Autodesk Fusion 360 part; units mm, degrees
note: some values were not read from the file. Chosen so that the rebuilt part matches the saved one: which bodies a step acts on. Set by a fixed rule: which sketch regions a step uses.
(part 5 of 5)
sketch "Sketch3 (7)" plane through (0, 0, -49) normal (0, 0, -1) x (1, 0, 0) in component "backing_ply"
  circle A0 centre (-129.840277, 129.840277) radius 1.6
  circle A1 centre (129.840277, -129.840277) radius 1.6
  circle A2 centre (129.840277, 129.840277) radius 1.6
  circle A3 centre (-129.840277, -129.840277) radius 1.6
  line L0 (143.5, -143.5) -> (143.5, 143.5)
  line L1 (143.5, 143.5) -> (-143.5, 143.5)
  line L2 (-143.5, 143.5) -> (-143.5, -143.5)
  line L3 (-143.5, -143.5) -> (143.5, -143.5)
  circle A4 centre (61.125, 122.25) radius 1.6
  line L4 (53.825, 131.25) -> (53.825, 122.25)
  arc A5 (53.825, 122.25) -> (68.425, 122.25) centre (61.125, 122.25) ccw
  line L5 (68.425, 122.25) -> (68.425, 131.25)
  arc A6 (67.425, 130.25) -> (68.425, 131.25) centre (67.425, 131.25) ccw
  line L6 (67.425, 130.25) -> (54.825, 130.25)
  arc A7 (53.825, 131.25) -> (54.825, 130.25) centre (54.825, 131.25) ccw
  circle A8 centre (122.25, 61.125) radius 1.6
  line L7 (122.25, 53.825) -> (131.25, 53.825)
  arc A9 (130.25, 54.825) -> (131.25, 53.825) centre (131.25, 54.825) ccw
  line L8 (130.25, 54.825) -> (130.25, 67.425)
  arc A10 (131.25, 68.425) -> (130.25, 67.425) centre (131.25, 67.425) ccw
  line L9 (131.25, 68.425) -> (122.25, 68.425)
  arc A11 (122.25, 68.425) -> (122.25, 53.825) centre (122.25, 61.125) ccw
  line L10 (69.3375, -105.4375) -> (99.8375, -105.4375)
  arc A12 (99.8375, -105.4375) -> (99.8375, -94.2375) centre (99.8375, -99.8375) ccw
  line L11 (99.8375, -94.2375) -> (69.3375, -94.2375)
  arc A13 (69.3375, -94.2375) -> (69.3375, -105.4375) centre (69.3375, -99.8375) ccw
  line L12 (69.3375, -99.8375) -> (99.8375, -99.8375) construction
  line L13 (94.8375, -96.2375) -> (74.3375, -96.2375)
  line L14 (74.3375, -96.2375) -> (74.3375, -103.4375)
  line L15 (74.3375, -103.4375) -> (94.8375, -103.4375)
  line L16 (94.8375, -103.4375) -> (94.8375, -96.2375)
  line L17 (94.8375, -96.2375) -> (74.3375, -103.4375) construction
  line L18 (74.3375, -96.2375) -> (94.8375, -103.4375) construction
  circle A14 centre (122.25, -61.125) radius 1.6
  line L19 (131.25, -53.825) -> (122.25, -53.825)
  arc A15 (122.25, -53.825) -> (122.25, -68.425) centre (122.25, -61.125) ccw
  line L20 (122.25, -68.425) -> (131.25, -68.425)
  arc A16 (130.25, -67.425) -> (131.25, -68.425) centre (131.25, -67.425) ccw
  line L21 (130.25, -67.425) -> (130.25, -54.825)
  arc A17 (131.25, -53.825) -> (130.25, -54.825) centre (131.25, -54.825) ccw
  circle A18 centre (61.125, -122.25) radius 1.6
  line L22 (53.825, -122.25) -> (53.825, -131.25)
  arc A19 (54.825, -130.25) -> (53.825, -131.25) centre (54.825, -131.25) ccw
  line L23 (54.825, -130.25) -> (67.425, -130.25)
  arc A20 (68.425, -131.25) -> (67.425, -130.25) centre (67.425, -131.25) ccw
  line L24 (68.425, -131.25) -> (68.425, -122.25)
  arc A21 (68.425, -122.25) -> (53.825, -122.25) centre (61.125, -122.25) ccw
  line L25 (96.8375, -101.569551) -> (99.8375, -103.301602)
  line L26 (99.8375, -103.301602) -> (102.8375, -101.569551)
  line L27 (102.8375, -101.569551) -> (102.8375, -98.105449)
  line L28 (102.8375, -98.105449) -> (99.8375, -96.373398)
  line L29 (99.8375, -96.373398) -> (96.8375, -98.105449)
  line L30 (96.8375, -98.105449) -> (96.8375, -101.569551)
  line L31 (72.3375, -98.105449) -> (69.3375, -96.373398)
  line L32 (69.3375, -96.373398) -> (66.3375, -98.105449)
  line L33 (66.3375, -98.105449) -> (66.3375, -101.569551)
  line L34 (66.3375, -101.569551) -> (69.3375, -103.301602)
  line L35 (69.3375, -103.301602) -> (72.3375, -101.569551)
  line L36 (72.3375, -101.569551) -> (72.3375, -98.105449)
  line L37 (69.3375, -105.5375) -> (99.8375, -105.5375)
  arc A22 (99.8375, -105.5375) -> (99.8375, -94.1375) centre (99.8375, -99.8375) ccw
  line L38 (99.8375, -94.1375) -> (69.3375, -94.1375)
  arc A23 (69.3375, -94.1375) -> (69.3375, -105.5375) centre (69.3375, -99.8375) ccw
  circle A24 centre (-122.25, -61.125) radius 1.6
  line L39 (-122.25, -53.825) -> (-131.25, -53.825)
  arc A25 (-130.25, -54.825) -> (-131.25, -53.825) centre (-131.25, -54.825) ccw
  line L40 (-130.25, -54.825) -> (-130.25, -67.425)
  arc A26 (-131.25, -68.425) -> (-130.25, -67.425) centre (-131.25, -67.425) ccw
  line L41 (-131.25, -68.425) -> (-122.25, -68.425)
  arc A27 (-122.25, -68.425) -> (-122.25, -53.825) centre (-122.25, -61.125) ccw
  circle A28 centre (-61.125, -122.25) radius 1.6
  line L42 (-53.825, -131.25) -> (-53.825, -122.25)
  arc A29 (-53.825, -122.25) -> (-68.425, -122.25) centre (-61.125, -122.25) ccw
  line L43 (-68.425, -122.25) -> (-68.425, -131.25)
  arc A30 (-67.425, -130.25) -> (-68.425, -131.25) centre (-67.425, -131.25) ccw
  line L44 (-67.425, -130.25) -> (-54.825, -130.25)
  arc A31 (-53.825, -131.25) -> (-54.825, -130.25) centre (-54.825, -131.25) ccw
  line L45 (-131.25, -68.425) -> (-68.425, -131.25) construction
  circle A32 centre (-99.8375, -99.8375) radius 5.35
  line L46 (-75, 143.5) -> (-75, -143.5) construction
  line L47 (75, 143.5) -> (75, -143.5) construction
  line L48 (-75, 108.5) -> (75, 108.5) construction
  line L49 (-75, 88.5) -> (75, 88.5) construction
  line L50 (-75, 58.5) -> (75, 58.5) construction
  circle A33 centre (75, 108.5) radius 5
  circle A34 centre (75, 58.5) radius 5
  line L51 (70.285955, 60.166667) -> (75, 73.5)
  line L52 (75, 73.5) -> (79.714045, 60.166667)
  circle A35 centre (75, 88.5) radius 5 construction
  circle A36 centre (75, 93.5) radius 2.5
  circle A37 centre (75, 83.5) radius 2.5
  line L53 (0, 108.5) -> (0, 58.5) construction
  circle A38 centre (-75, 108.5) radius 5
  circle A39 centre (-75, 93.5) radius 2.5
  circle A40 centre (-75, 83.5) radius 2.5
  line L54 (-75, 73.5) -> (-79.714045, 60.166667)
  line L55 (-70.285955, 60.166667) -> (-75, 73.5)
  circle A41 centre (-75, 58.5) radius 5
  line L56 (0, 108.5) -> (75, 58.5) construction
  line L57 (37.5, 83.5) -> (37.5, 108.5) construction
  circle A42 centre (0, 108.5) radius 5
  circle A43 centre (0, 93.5) radius 2.5
  circle A44 centre (0, 83.5) radius 2.5
  line L58 (4.714045, 60.166667) -> (0, 73.5)
  line L59 (0, 73.5) -> (-4.714045, 60.166667)
  circle A45 centre (0, 58.5) radius 5
  line L60 (68.425, -131.25) -> (131.25, -68.425) construction
  point P0 (84.5875, -99.8375)
  point P1 (84.5875, -99.8375)
  point P2 (84.5875, -99.8375)
  point P3 (84.5875, -99.8375)
  point P4 (99.8375, -99.8375)
  point P5 (69.3375, -99.8375)
  point P6 (0, 143.5)
  point P7 (75, 103.5)
  point P8 (99.8375, -99.8375)
  point P9 (72.3375, -99.8375)
  dimension "d403" = 7.2
  dimension "d404" = 20.5
  dimension "d405" = 2
  dimension "d406" = 3
  dimension "d407" = 3
  dimension "d408" = 2
  dimension "d409" = 0.1
  dimension "d410" = 10.7
  dimension "d413" = 150
  dimension "d414" = 75
  dimension "d415" = 10
  dimension "d416" = 10
  dimension "d417" = 10
  dimension "d418" = 15
  dimension "d419" = 5
  dimension "d420" = 5
  dimension "d421" = 35
  dimension "d422" = 50
  dimension "d424" = 30
  dimension "d425" = 15
  constraint tangent L10 A12
  constraint tangent A12 L11
  constraint parallel L10 L11
  constraint tangent L11 A13
  constraint tangent L10 A13
  constraint horizontal L12
  constraint coincident P3 P2
  constraint midpoint L12 P3
  constraint horizontal L13
  constraint perpendicular L13 L14
  constraint parallel L13 L15
  constraint parallel L14 L16
  constraint coincident L17 P3
  constraint coincident L18 P3
  constraint coincident P8 P4
  constraint coincident P5 A13.centre
  constraint coincident A26.start L41.start
  constraint coincident L43.end A30.end
  constraint midpoint L45 A32.centre
  constraint coincident L1 L46.start
  constraint coincident L3 L46.end
  constraint perpendicular L3 L46
  constraint coincident L1 L47.start
  constraint coincident L3 L47.end
  constraint perpendicular L3 L47
  constraint midpoint L1 P6
  constraint coincident L46 L48.start
  constraint coincident L47 L48.end
  constraint perpendicular L47 L48
  constraint coincident L46 L49.start
  constraint coincident L47 L49.end
  constraint perpendicular L47 L49
  constraint coincident L46 L50.start
  constraint coincident L47 L50.end
  constraint perpendicular L47 L50
  constraint coincident L48.end A33.centre
  constraint coincident L50.end A34.centre
  constraint coincident L47 L51.end
  constraint tangent A34 L51
  constraint tangent A34 L52
  constraint coincident L49.end A35.centre
  constraint coincident A35 A36.centre
  constraint coincident L47 A36.centre
  constraint coincident L47 A37.centre
  constraint coincident A35 A37.centre
  constraint coincident A33 P7
  constraint coincident L47 P7
  constraint midpoint L48 L53.start
  constraint midpoint L50 L53.end
  constraint symmetric A33 L53 A38
  constraint symmetric A34 L53 A41
  constraint symmetric L51.end L53 L54.start
  constraint symmetric A36 L53 A39
  constraint symmetric A37 L53 A40
  constraint midpoint L56 L57.start
  constraint coincident L48 L57.end
  constraint perpendicular L48 L57
  constraint symmetric A33 L57 A42
  constraint symmetric A34 L57 A45
  constraint symmetric L51.end L57 L58.end
  constraint symmetric A36 L57 A43
  constraint symmetric A37 L57 A44
  constraint coincident A20.start L24.start
  constraint coincident L20.end A16.end
  constraint midpoint L60 P8
  constraint midpoint L36 P9
  constraint coincident L12 P9
  measures "d403" distance of L13.start L15.end
  measures "d404" distance of L14 L16
  measures "d405" distance of L11 L13
  measures "d406" distance of P8 L30
  measures "d407" distance of P5 L36
  measures "d408" distance of L16 L30
  measures "d410" diameter of A32
  measures "d413" distance of L46 L47
  measures "d414" distance of L47 P6
  measures "d415" diameter of A33
  measures "d416" diameter of A34
  measures "d417" diameter of A35
  measures "d418" distance of L50.end L51.end
  measures "d419" diameter of A36
  measures "d420" diameter of A37
  measures "d421" distance of L1 L48
  measures "d422" distance of L48 L50
  measures "d424" distance of L51.end P7
  measures "d425" distance of L49.end P7
extrude "Extrude3''''''" cut sketch "Sketch3 (7)" against normal blind 10 contours L10 A12 L11 A13 | L13 L14 L15 L16 | L25 L26 L27 L28 L29 L30 | L31 L32 L33 L34 L35 L36 | L37 A22 L38 A23 | A32 | A33 | A34 | A34 L51 L52 | A36 | A37 | A38 | A39 | A40 | L54 L55 A41 | A41 | A42 | A43 | A44 | L58 L59 A45 | A45 picked at (88.004167, -94.904167) picked at (81.170833, -98.6375) picked at (100.8375, -100.41485) picked at (68.3375, -99.26015) picked at (79.504167, -105.470833) picked at (-98.230772, -100.611259) picked at (76.446185, 108.980285) picked at (75.428311, 60.054771) picked at (75, 66.824599) picked at (76.760267, 93.305637) picked at (76.760267, 83.305637) picked at (-73.553815, 108.980285) picked at (-73.239733, 93.305637) picked at (-73.239733, 83.305637) picked at (-75, 66.824599) picked at (-71.930398, 57.383078) picked at (-1.574006, 108.257145) picked at (-0.062275, 94.331003) picked at (-1.856006, 82.886176) picked at (0, 66.824599) picked at (1.18045, 60.362306) bodies 49 in component "backing_ply"
sketch "Sketch1 (6)" plane through (0, 0, -49) normal (0, 0, -1) x (1, 0, 0) in component "programming-port_3d"
  circle A0 centre (75, 83.5) radius 2.5
  circle A1 centre (0, 93.5) radius 2.5
  circle A2 centre (-75, 83.5) radius 2.5
  circle A3 centre (-99.8375, -99.8375) radius 5.35
  circle A4 centre (-75, 93.5) radius 2.5
  circle A5 centre (0, 83.5) radius 2.5
  circle A6 centre (75, 93.5) radius 2.5
  line L0 (75, 73.5) -> (79.714045, 60.166667)
  arc A7 (70.285955, 60.166667) -> (79.714045, 60.166667) centre (75, 58.5) ccw
  line L1 (70.285955, 60.166667) -> (75, 73.5)
  circle A8 centre (0, 108.5) radius 5
  line L2 (-75, 73.5) -> (-70.285955, 60.166667)
  arc A9 (-79.714045, 60.166667) -> (-70.285955, 60.166667) centre (-75, 58.5) ccw
  line L3 (-79.714045, 60.166667) -> (-75, 73.5)
  line L4 (99.8375, -105.5375) -> (69.3375, -105.5375)
  arc A10 (69.3375, -94.1375) -> (69.3375, -105.5375) centre (69.3375, -99.8375) ccw
  line L5 (69.3375, -94.1375) -> (99.8375, -94.1375)
  arc A11 (99.8375, -105.5375) -> (99.8375, -94.1375) centre (99.8375, -99.8375) ccw
  circle A12 centre (-75, 108.5) radius 5
  line L6 (0, 73.5) -> (4.714045, 60.166667)
  arc A13 (-4.714045, 60.166667) -> (4.714045, 60.166667) centre (0, 58.5) ccw
  line L7 (-4.714045, 60.166667) -> (0, 73.5)
  circle A14 centre (75, 108.5) radius 5
  circle A15 centre (-129.840277, 129.840277) radius 1.6
  circle A16 centre (129.840277, -129.840277) radius 1.6
  circle A17 centre (129.840277, 129.840277) radius 1.6
  circle A18 centre (-129.840277, -129.840277) radius 1.6
  line L8 (143.5, -143.5) -> (143.5, 143.5)
  line L9 (143.5, 143.5) -> (-143.5, 143.5)
  line L10 (-143.5, 143.5) -> (-143.5, -143.5)
  line L11 (-143.5, -143.5) -> (143.5, -143.5)
  arc A19 (69.3375, -94.2375) -> (69.3375, -105.4375) centre (69.3375, -99.8375) ccw
  line L12 (99.8375, -94.2375) -> (69.3375, -94.2375)
  line L13 (69.3375, -96.373398) -> (66.3375, -98.105449)
  line L14 (72.3375, -98.105449) -> (69.3375, -96.373398)
  line L15 (66.3375, -98.105449) -> (66.3375, -101.569551)
  line L16 (66.3375, -101.569551) -> (69.3375, -103.301602)
  line L17 (69.3375, -103.301602) -> (72.3375, -101.569551)
  line L18 (72.3375, -101.569551) -> (72.3375, -98.105449)
  line L19 (94.8375, -96.2375) -> (74.3375, -96.2375)
  line L20 (74.3375, -96.2375) -> (74.3375, -103.4375)
  line L21 (74.3375, -103.4375) -> (94.8375, -103.4375)
  line L22 (94.8375, -103.4375) -> (94.8375, -96.2375)
  line L23 (99.8375, -96.373398) -> (96.8375, -98.105449)
  line L24 (102.8375, -98.105449) -> (99.8375, -96.373398)
  line L25 (102.8375, -101.569551) -> (102.8375, -98.105449)
  line L26 (99.8375, -103.301602) -> (102.8375, -101.569551)
  line L27 (96.8375, -101.569551) -> (99.8375, -103.301602)
  line L28 (96.8375, -98.105449) -> (96.8375, -101.569551)
  arc A20 (99.8375, -105.4375) -> (99.8375, -94.2375) centre (99.8375, -99.8375) ccw
  line L29 (69.3375, -105.4375) -> (99.8375, -105.4375)
  line L30 (69.3375, -106.9375) -> (99.8375, -106.9375)
  arc A21 (99.8375, -106.9375) -> (99.8375, -92.7375) centre (99.8375, -99.8375) ccw
  line L31 (99.8375, -92.7375) -> (69.3375, -92.7375)
  arc A22 (69.3375, -92.7375) -> (69.3375, -106.9375) centre (69.3375, -99.8375) ccw
  line L32 (74.3375, -96.2375) -> (94.8375, -103.4375) construction
  line L33 (94.8375, -96.2375) -> (74.3375, -103.4375) construction
  line L34 (78.4875, -103.0875) -> (90.6875, -103.0875)
  arc A23 (90.6875, -103.0875) -> (90.6875, -96.5875) centre (90.6875, -99.8375) ccw
  line L35 (90.6875, -96.5875) -> (78.4875, -96.5875)
  arc A24 (78.4875, -96.5875) -> (78.4875, -103.0875) centre (78.4875, -99.8375) ccw
  line L36 (78.4875, -99.8375) -> (90.6875, -99.8375) construction
  point P0 (84.5875, -99.8375)
  dimension "d426" = 1.5
  dimension "d427" = 12.2
  dimension "d428" = 6.5
  constraint coincident L19.end L20.start
  constraint coincident L21.end L22.start
  constraint coincident L19.start L22.end
  constraint coincident L20.end L21.start
  constraint tangent L34 A23
  constraint tangent A23 L35
  constraint parallel L34 L35
  constraint tangent L35 A24
  constraint tangent L34 A24
  constraint horizontal L36
  constraint midpoint L32 P0
  constraint midpoint L36 P0
  measures "d427" distance of A23.end L35.end
  measures "d428" distance of L34 L35
extrude "Extrude1'''''''" add sketch "Sketch1 (6)" along normal blind 2 separate body contours L4 A10 L5 A11 | A19 L12 A20 L29 | L13 L14 L15 L16 L17 L18 | L19 L20 L21 L22 | L23 L24 L25 L26 L27 L28 | L30 A21 L31 A22 picked at (79.504167, -105.470833) picked at (81.170833, -94.904167) picked at (68.3375, -99.26015) picked at (94.534471, -99.756542) picked at (100.8375, -99.26015) picked at (89.670833, -93.204167) makes body 50 in component "programming-port_3d"
fillet "Fillet1''" radius 1.5 4 edges at (93.9375, 99.8375, -51) (84.5875, 103.0875, -51) (75.2375, 99.8375, -51) (84.5875, 96.5875, -51) on bodies 50 in component "programming-port_3d"
extrude "Extrude2'''''" add sketch "Sketch1 (6)" against normal blind 3 contours A19 L12 A20 L29 picked at (81.170833, -94.904167) bodies 50 in component "programming-port_3d"
sketch "Sketch4 (4)" plane through (0, 0, -46) normal (0, 0, 1) x (-1, 0, 0) in component "programming-port_3d"
  line L0 (-72.3375, -101.569551) -> (-72.3375, -98.105449)
  line L1 (-72.3375, -98.105449) -> (-69.3375, -96.373398)
  line L2 (-69.3375, -96.373398) -> (-66.3375, -98.105449)
  line L3 (-66.3375, -98.105449) -> (-66.3375, -101.569551)
  line L4 (-66.3375, -101.569551) -> (-69.3375, -103.301602)
  line L5 (-69.3375, -103.301602) -> (-72.3375, -101.569551)
  line L6 (-94.8375, -103.4375) -> (-94.8375, -96.2375)
  line L7 (-94.8375, -96.2375) -> (-74.3375, -96.2375)
  line L8 (-74.3375, -96.2375) -> (-74.3375, -103.4375)
  line L9 (-74.3375, -103.4375) -> (-94.8375, -103.4375)
  line L10 (-96.8375, -98.105449) -> (-96.8375, -101.569551)
  line L11 (-96.8375, -101.569551) -> (-99.8375, -103.301602)
  line L12 (-99.8375, -103.301602) -> (-102.8375, -101.569551)
  line L13 (-102.8375, -101.569551) -> (-102.8375, -98.105449)
  line L14 (-102.8375, -98.105449) -> (-99.8375, -96.373398)
  line L15 (-99.8375, -96.373398) -> (-96.8375, -98.105449)
  line L16 (-99.8375, -105.4375) -> (-69.3375, -105.4375)
  arc A0 (-69.3375, -105.4375) -> (-69.3375, -94.2375) centre (-69.3375, -99.8375) ccw
  line L17 (-69.3375, -94.2375) -> (-99.8375, -94.2375)
  arc A1 (-99.8375, -94.2375) -> (-99.8375, -105.4375) centre (-99.8375, -99.8375) ccw
  line L18 (-72.3375, -101.569551) -> (-69.3375, -103.301602)
  line L19 (-69.3375, -103.301602) -> (-66.3375, -101.569551)
  line L20 (-66.3375, -101.569551) -> (-66.3375, -98.105449)
  line L21 (-66.3375, -98.105449) -> (-69.3375, -96.373398)
  line L22 (-69.3375, -96.373398) -> (-72.3375, -98.105449)
  line L23 (-72.3375, -98.105449) -> (-72.3375, -101.569551)
  line L24 (-96.8375, -98.105449) -> (-99.8375, -96.373398)
  line L25 (-99.8375, -96.373398) -> (-102.8375, -98.105449)
  line L26 (-102.8375, -98.105449) -> (-102.8375, -101.569551)
  line L27 (-102.8375, -101.569551) -> (-99.8375, -103.301602)
  line L28 (-99.8375, -103.301602) -> (-96.8375, -101.569551)
  line L29 (-96.8375, -101.569551) -> (-96.8375, -98.105449)
  line L30 (-99.8375, -96.373398) -> (-99.8375, -103.301602) construction
  line L31 (-96.8375, -98.105449) -> (-102.8375, -101.569551) construction
  line L32 (-69.3375, -96.373398) -> (-69.3375, -103.301602) construction
  line L33 (-66.3375, -98.105449) -> (-72.3375, -101.569551) construction
  circle A2 centre (-69.3375, -99.8375) radius 1.6
  circle A3 centre (-99.8375, -99.8375) radius 1.6
  dimension "d437" = 3.2
  dimension "d438" = 3.2
  constraint concentric A0 A2
  constraint concentric A1 A3
  measures "d437" diameter of A2
  measures "d438" diameter of A3
extrude "Extrude3'''''''" add sketch "Sketch4 (4)" along normal blind 2 contours L0 L1 L2 L3 L4 L5 L18 L19 L20 L21 L22 L23 | L10 L11 L12 L13 L14 L15 L24 L25 L26 L27 L28 L29 | L16 A0 L17 A1 picked at (-66.804167, -99.8375) picked at (-102.370833, -99.8375) picked at (-88.004167, -94.904167) bodies 50 in component "programming-port_3d"
sketch "Sketch1 (7)" plane through (0, 0, -44) normal (0, 0, 1) x (-1, 0, 0) in component "back"
  line L0 (-74.3375, -96.2375) -> (-74.3375, -103.4375)
  line L1 (-74.3375, -103.4375) -> (-94.8375, -103.4375)
  line L2 (-94.8375, -103.4375) -> (-94.8375, -96.2375)
  line L3 (-94.8375, -96.2375) -> (-74.3375, -96.2375)
  circle A0 centre (-69.3375, -99.8375) radius 1.6
  circle A1 centre (-99.8375, -99.8375) radius 1.6
  arc A2 (-99.8375, -94.2375) -> (-99.8375, -105.4375) centre (-99.8375, -99.8375) ccw
  line L4 (-99.8375, -105.4375) -> (-69.3375, -105.4375)
  arc A3 (-69.3375, -105.4375) -> (-69.3375, -94.2375) centre (-69.3375, -99.8375) ccw
  line L5 (-69.3375, -94.2375) -> (-99.8375, -94.2375)
  line L6 (-94.8375, -96.2375) -> (-74.3375, -103.4375) construction
  line L7 (-74.3375, -96.2375) -> (-94.8375, -103.4375) construction
  line L8 (-79.8375, -96.2375) -> (-89.3375, -96.2375) construction
  line L9 (-89.3375, -96.2375) -> (-89.3375, -103.4375)
  line L10 (-89.3375, -103.4375) -> (-79.8375, -103.4375) construction
  line L11 (-79.8375, -103.4375) -> (-79.8375, -96.2375)
  line L12 (-79.8375, -96.2375) -> (-89.3375, -103.4375) construction
  line L13 (-89.3375, -96.2375) -> (-79.8375, -103.4375) construction
  line L14 (-74.6375, -103.1375) -> (-94.5375, -103.1375)
  line L15 (-94.5375, -103.1375) -> (-94.5375, -96.5375)
  line L16 (-94.5375, -96.5375) -> (-74.6375, -96.5375)
  line L17 (-74.6375, -96.5375) -> (-74.6375, -103.1375)
  point P0 (-84.5875, -99.8375)
  dimension "d439" = 9.5
  dimension "d440" = 0.3
  constraint coincident L2.end L3.start
  constraint coincident L0.end L1.start
  constraint coincident L0.start L3.end
  constraint coincident L1.end L2.start
  constraint horizontal L8
  constraint perpendicular L8 L9
  constraint parallel L8 L10
  constraint parallel L9 L11
  constraint coincident L12 P0
  constraint coincident L13 P0
  constraint coincident L3 L8.start
  constraint midpoint L6 P0
  measures "d439" distance of L8.start L8.end
extrude "Extrude1''''''''" add sketch "Sketch1 (7)" against normal blind 3.4 separate body contours L11 L14 L16 L17 | L9 L14 L15 L16 picked at (-76.370833, -98.7375) picked at (-91.070833, -98.7375) makes body 51 at (91.070833, 98.7375, -44) makes body 52 at (76.370833, 98.7375, -44) in component "back"
extrude "Extrude2''''''" add sketch "Sketch1 (7)" along normal blind 5 contours L0 L1 L3 L11 L14 L16 L17 | L1 L2 L3 L9 L14 L15 L16 | L11 L14 L16 L17 | L9 L14 L15 L16 | A2 L4 A3 L5 picked at (-74.4375, -98.7375) picked at (-94.7375, -100.9375) picked at (-76.370833, -98.7375) picked at (-91.070833, -98.7375) picked at (-95.970833, -99.8375) bodies 51 52 in component "back"
fillet "Fillet1'''" radius 2 2 edges at (89.3375, 99.8375, -47.4) (79.8375, 99.8375, -47.4) on bodies 51 in component "back"
sketch "Sketch2 (6)" plane through (0, 0, -39) normal (0, 0, 1) x (-1, 0, 0) in component "back"
  line L0 (-89.3375, -103.4375) -> (-89.3375, -96.2375)
  line L1 (-89.3375, -96.2375) -> (-79.8375, -96.2375)
  line L2 (-79.8375, -96.2375) -> (-79.8375, -103.4375)
  line L3 (-79.8375, -103.4375) -> (-89.3375, -103.4375)
  circle A0 centre (-99.8375, -99.8375) radius 1.6
  circle A1 centre (-69.3375, -99.8375) radius 1.6
  line L4 (-69.3375, -94.2375) -> (-99.8375, -94.2375)
  arc A2 (-99.8375, -94.2375) -> (-99.8375, -105.4375) centre (-99.8375, -99.8375) ccw
  line L5 (-99.8375, -105.4375) -> (-69.3375, -105.4375)
  arc A3 (-69.3375, -105.4375) -> (-69.3375, -94.2375) centre (-69.3375, -99.8375) ccw
  arc A4 (-69.3375, -106.9375) -> (-69.3375, -92.7375) centre (-69.3375, -99.8375) ccw
  line L6 (-69.3375, -92.7375) -> (-99.8375, -92.7375)
  arc A5 (-99.8375, -92.7375) -> (-99.8375, -106.9375) centre (-99.8375, -99.8375) ccw
  line L7 (-99.8375, -106.9375) -> (-69.3375, -106.9375)
  arc A6 (-99.8375, -94.2375) -> (-99.8375, -105.4375) centre (-99.8375, -99.8375) ccw
  line L8 (-99.8375, -94.2375) -> (-69.3375, -94.2375)
  arc A7 (-69.3375, -105.4375) -> (-69.3375, -94.2375) centre (-69.3375, -99.8375) ccw
  line L9 (-69.3375, -105.4375) -> (-99.8375, -105.4375)
extrude "Extrude3''''''''" add sketch "Sketch2 (6)" against normal blind 7 contours A4 L6 A5 L7 picked at (-89.670833, -106.4375) bodies 51 in component "back"
sketch "Sketch3 (8)" plane through (0, 0, -46) normal (0, 0, -1) x (1, 0, 0) in component "back"
  arc A0 (99.8375, -105.4375) -> (99.8375, -94.2375) centre (99.8375, -99.8375) ccw
  line L0 (99.8375, -105.4375) -> (69.3375, -105.4375)
  arc A1 (69.3375, -94.2375) -> (69.3375, -105.4375) centre (69.3375, -99.8375) ccw
  line L1 (69.3375, -94.2375) -> (99.8375, -94.2375)
  line L2 (69.3375, -106.9375) -> (99.8375, -106.9375)
  arc A2 (99.8375, -106.9375) -> (99.8375, -92.7375) centre (99.8375, -99.8375) ccw
  line L3 (99.8375, -92.7375) -> (69.3375, -92.7375)
  arc A3 (69.3375, -92.7375) -> (69.3375, -106.9375) centre (69.3375, -99.8375) ccw
  arc A4 (69.3375, -92.7375) -> (69.3375, -106.9375) centre (69.3375, -99.8375) ccw
  line L4 (69.3375, -92.7375) -> (99.8375, -92.7375)
  arc A5 (99.8375, -106.9375) -> (99.8375, -92.7375) centre (99.8375, -99.8375) ccw
  line L5 (99.8375, -106.9375) -> (69.3375, -106.9375)
  arc A6 (99.8375, -105.4375) -> (99.8375, -94.2375) centre (99.8375, -99.8375) ccw
  line L6 (99.8375, -94.2375) -> (69.3375, -94.2375)
  arc A7 (69.3375, -94.2375) -> (69.3375, -105.4375) centre (69.3375, -99.8375) ccw
  line L7 (69.3375, -105.4375) -> (99.8375, -105.4375)
  arc A8 (99.8375, -105.7375) -> (99.8375, -93.9375) centre (99.8375, -99.8375) ccw
  line L8 (69.3375, -93.9375) -> (99.8375, -93.9375)
  arc A9 (69.3375, -93.9375) -> (69.3375, -105.7375) centre (69.3375, -99.8375) ccw
  line L9 (99.8375, -105.7375) -> (69.3375, -105.7375)
  dimension "d449" = -0.3
extrude "Extrude4'''" cut sketch "Sketch3 (8)" against normal blind 2 contours A8 L8 A9 L9 picked at (89.670833, -105.6375) bodies 51 in component "back"
component "clock-face_black-polypropylene" placed x (1, 0, 0) y (0, 1, 0) z (0, 0, 1) at (0, 0, 0)
component "cover_clear-acrylic" placed x (1, 0, 0) y (0, 1, 0) z (0, 0, 1) at (0, 0, 0)
component "diffusion_white-acrylic" placed x (1, 0, 0) y (0, 1, 0) z (0, 0, 1) at (0, 0, 0)
component "grid-frame_3d" placed x (1, 0, 0) y (0, 1, 0) z (0, 0, 1) at (0, 0, 0)
component "led-pannel-frame_ply" placed x (1, 0, 0) y (0, 1, 0) z (0, 0, 1) at (0, 0, 0)
component "grid_3d" placed x (1, 0, 0) y (0, 1, 0) z (0, 0, 1) at (0, 0, 0)
component "frame-brackets_3d" placed x (1, 0, 0) y (0, 1, 0) z (0, 0, 1) at (0, 0, 0)
component "sides" placed x (1, 0, 0) y (0, 1, 0) z (0, 0, 1) at (0, 0, 0)
component "backing_ply" placed x (1, 0, 0) y (0, 1, 0) z (0, 0, 1) at (0, 0, 0)
component "bolt-holder_3d" placed x (1, 0, 0) y (0, 1, 0) z (0, 0, 1) at (0, 0, 0)
component "programming-port_3d" placed x (1, 0, 0) y (0, 1, 0) z (0, 0, 1) at (0, 0, 0)
component "spacer" placed x (1, 0, 0) y (0, 1, 0) z (0, 0, 1) at (0, 0, 0) in component "grid-frame_3d"
component "corner-bracket_3d" placed x (1, 0, 0) y (0, 1, 0) z (0, 0, 1) at (0, 0, 0) in component "frame-brackets_3d"
component "edge-bracket_3d" placed x (1, 0, 0) y (0, 1, 0) z (0, 0, 1) at (0, 0, 0) in component "frame-brackets_3d"
component "back" placed x (1, 0, 0) y (0, 1, 0) z (0, 0, 1) at (0, 0, 0) in component "programming-port_3d"
equation "d123 = d121"
equation "d124 = d123"
equation "d128 = d127"
equation "d162 = d161 + 5 * 2 mm"
equation "d172 = d164 / 2"
equation "d174 = d163"
equation "d175 = d164 / 2"
equation "d189 = d186"
equation "d190 = d188"
equation "d206 = d205"
equation "d216 = d214 / 4"
equation "d217 = -d164 * 0.75"
equation "d231 = d230 - 0.5 mm"
equation "d232 = ( d230 - d231 ) / 2"
equation "d241 = d164"
equation "d247 = -( d164 / 2 ) - 0.25 mm"
equation "d283 = d282"
equation "d284 = d282"
equation "d290 = d289"
equation "d292 = -10 mm + 3 mm"
equation "d295 = d294"
equation "d297 = -10 mm + 3 mm"
equation "d299 = -25.00 mm + 4 mm"
equation "d306 = -34.142 mm - ( ( 7 / 2 ) * 1 mm )"
equation "d312 = ( 6 / 2 ) * 1 mm"
equation "d325 = ( 6 / 2 ) * 1 mm"
equation "d339 = -10 mm + 3 mm"
equation "d341 = ( 6.2 / 2 ) * 1 mm"
equation "d355 = d354"
equation "d356 = d357 / 5"
equation "d361 = d357 - d356"
equation "d370 = d369 / 2"
equation "d403 = 6.7 mm + 0.5 mm"
equation "d404 = 20 mm + 0.5 mm"
equation "d408 = d405"
equation "d414 = d413 / 2"
equation "d425 = d424 / 2"
equation "d441 = -5.00 mm + 1.6 mm"
equation "d443 = -5.00 mm + 10 mm"
named bodies: "bottom-side_black-acrylic", "side_black-acrylic", "side_black-acrylic (1)", "side_black-acrylic (2)"
